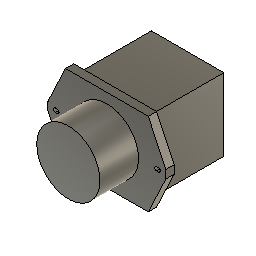
df5fb8b6-cb67-4064-a8af-0fe8c923339c (Autodesk Fusion 360 design; units mm, degrees)
Autodesk Fusion 360 part; units mm, degrees
note: some values were not read from the file. Set by a fixed rule: which sketch regions a step uses.
sketch "Sketch1" plane through (0, 0, 0) normal (0, 1, 0) x (1, 0, 0)
  line L0 (-73.5, -97.2411) -> (-23.5, -97.2411)
  line L1 (-72.5, -97.2411) -> (-24.5, -97.2411) construction
  line L2 (-77, -97.2411) -> (-20, -97.2411) construction
  line L3 (-48.5, -117.2411) -> (-48.5, -77.2411)
  line L4 (-23.5, -96.3461) -> (-24.5, -96.3461)
  arc A0 (-24.5, -96.3461) -> (-24.5, -98.1361) centre (-24.5, -97.2411) ccw
  line L5 (-24.5, -98.1361) -> (-23.5, -98.1361)
  arc A1 (-23.5, -98.1361) -> (-23.5, -96.3461) centre (-23.5, -97.2411) ccw
  line L6 (-23.5, -97.2411) -> (-24.5, -97.2411) construction
  line L7 (-72.5, -96.3461) -> (-73.5, -96.3461)
  arc A2 (-73.5, -96.3461) -> (-73.5, -98.1361) centre (-73.5, -97.2411) ccw
  line L8 (-73.5, -98.1361) -> (-72.5, -98.1361)
  arc A3 (-72.5, -98.1361) -> (-72.5, -96.3461) centre (-72.5, -97.2411) ccw
  line L9 (-72.5, -97.2411) -> (-73.5, -97.2411) construction
  circle A4 centre (-48.5, -97.2411) radius 15.2574
  line L10 (-31, -114.7411) -> (-66, -114.7411)
  line L11 (-66, -114.7411) -> (-66, -79.7411)
  line L12 (-66, -79.7411) -> (-31, -79.7411)
  line L13 (-31, -79.7411) -> (-31, -114.7411)
  line L14 (-48.5, -114.7411) -> (-48.5, -79.7411) construction
  line L15 (-31, -97.2411) -> (-66, -97.2411) construction
  line L16 (-68.5, -117.2411) -> (-28.5, -117.2411)
  line L17 (-28.5, -117.2411) -> (-28.5, -77.2411) construction
  line L18 (-28.5, -77.2411) -> (-68.5, -77.2411)
  line L19 (-68.5, -77.2411) -> (-68.5, -117.2411) construction
  line L20 (-68.5, -97.2411) -> (-28.5, -97.2411) construction
  line L21 (-68.5, -117.2411) -> (-77, -99.2411)
  line L22 (-77, -99.2411) -> (-77, -97.2411)
  line L23 (-77, -97.2411) -> (-77, -95.2411)
  line L24 (-77, -95.2411) -> (-68.5, -77.2411)
  line L25 (-28.5, -117.2411) -> (-20, -99.2411)
  line L26 (-20, -99.2411) -> (-20, -97.2411)
  line L27 (-20, -97.2411) -> (-20, -95.2411)
  line L28 (-20, -95.2411) -> (-28.5, -77.2411)
  dimension "d1" = 50
  dimension "d2" = 48
  dimension "d3" = 57
  dimension "d4" = 40
  dimension "d5" = 1.79
  dimension "d6" = 1.79
  dimension "d7" = 35
  dimension "d8" = 35
  dimension "d9" = 40
  dimension "d10" = 40
  dimension "d11" = 4
  constraint horizontal L0
  constraint parallel L0 L1
  constraint horizontal L2
  constraint midpoint L1 L2
  constraint midpoint L0 L2
  constraint perpendicular L2 L3
  constraint midpoint L2 L3
  constraint tangent L4 A0
  constraint tangent A0 L5
  constraint parallel L4 L5
  constraint tangent L5 A1
  constraint tangent L4 A1
  constraint coincident L1.end A0.centre
  constraint parallel L0 L6
  constraint coincident L0.end A1.centre
  constraint tangent L7 A2
  constraint tangent A2 L8
  constraint parallel L7 L8
  constraint tangent L8 A3
  constraint tangent L7 A3
  constraint coincident L0.start A2.centre
  constraint parallel L0 L9
  constraint coincident L1.start A3.centre
  constraint midpoint L3 A4.centre
  constraint horizontal L10
  constraint vertical L11
  constraint horizontal L12
  constraint vertical L13
  constraint midpoint L10 L14.start
  constraint midpoint L12 L14.end
  constraint midpoint L13 L15.start
  constraint midpoint L11 L15.end
  constraint midpoint L0 L15
  constraint horizontal L16
  constraint vertical L17
  constraint horizontal L18
  constraint vertical L19
  constraint midpoint L19 L20.start
  constraint midpoint L17 L20.end
  constraint midpoint L1 L20
  constraint perpendicular L2 L23
  constraint equal L21 L24
  constraint equal L22 L23
  constraint symmetric L2.start L3 L2.end
  constraint symmetric L3 L16.start L16.end
  constraint symmetric L3 L18.end L17.end
  constraint symmetric L3 L21.end L25.end
  constraint symmetric L3 L23.end L27.end
  measures "d1" distance of L0.start L0.end
  measures "d2" distance of L1.start L1.end
  measures "d3" distance of L2.start L2.end
  measures "d4" distance of L3.start L3.end
  measures "d5" diameter of A0
  measures "d6" diameter of A2
  measures "d7" distance of L10.start L10.end
  measures "d8" distance of L10.start L12.end
  measures "d9" distance of L16.start L16.end
  measures "d10" distance of L16.start L18.end
  measures "d11" distance of L21.end L23.end
extrude "Extrude1" add sketch "Sketch1" along normal blind 35 contours L0 L3 A4 L11 L12 | L0 L3 A4 L10 L11 | L0 L3 A4 | L0 L3 A4 | L0 L3 A4 | L0 L3 A4 | L0 L3 A4 L12 L13 | L0 L3 A4 L10 L13
extrude "Extrude2" add sketch "Sketch1" against normal blind 4
extrude "Extrude3" add sketch "Sketch1" against normal blind 22.6 contours L0 L3 A4 | L0 L3 A4 | L0 L3 A4 | L0 L3 A4
equation "d16 = -26.6 mm + 4 mm"
